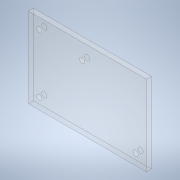
# Autodesk Inventor part: Template
Saved by Autodesk Inventor 2021 (Build 250183000, 183)
## iProperties
Created: 2021-05-20
Part Number: Template
Material: Polycarbonate, Clear
Document SubType Name: Modeling
Designer: maza168
Density: 1.2 g/cm^3
Appearance: Polycarbonate - Clear
Author: maza168
Autodesk Inventor part; units mm, degrees
ref_plane "YZ Plane" through (0, 0, 0) normal (1, 0, 0) x (0, 1, 0)
ref_plane "XZ Plane" through (0, 0, 0) normal (0, 1, 0) x (-1, 0, 0)
ref_plane "XY Plane" through (0, 0, 0) normal (0, 0, 1) x (1, 0, 0)
sketch "Sketch1" plane through (0, 0, 0) normal (0, 0, 1) x (1, 0, 0)
  line L0 (-110, 75) -> (110, 75)
  line L1 (110, 75) -> (110, -75)
  line L2 (110, -75) -> (-110, -75)
  line L3 (-110, -75) -> (-110, 75)
  line L4 (40, -10) -> (60, -10) construction
  line L5 (60, -10) -> (60, -30) construction
  line L6 (60, -30) -> (40, -30) construction
  line L7 (40, -30) -> (40, -10) construction
  line L8 (-67, 0) -> (-42, 0) construction
  line L9 (-42, 0) -> (-42, -30) construction
  line L10 (-42, -30) -> (-67, -30) construction
  line L11 (-67, -30) -> (-67, 0) construction
  circle A0 centre (-90, 55) radius 5
  circle A1 centre (-90, -55) radius 5
  circle A2 centre (90, -55) radius 5
  circle A3 centre (-10, 45) radius 5
  line L12 (-110, 75) -> (110, -75) construction
  line L13 (110, 75) -> (-110, -75) construction
  point P0 (0, 0)
  dimension "d0" = 220
  dimension "d1" = 150
  dimension "d2" = 110
  dimension "d3" = 75
  dimension "d4" = 20
  dimension "d5" = 20
  dimension "d6" = 10
  dimension "d7" = 40
  dimension "d8" = 10
  dimension "d9" = 90
  dimension "d10" = 55
  dimension "d11" = 10
  dimension "d12" = 10
  dimension "d13" = 10
  dimension "d14" = 55
  dimension "d15" = 42
  dimension "d16" = 30
  dimension "d17" = 25
  dimension "d18" = 0
  dimension "d19" = 90
  dimension "d20" = 45
  dimension "d21" = 10
  dimension "d22" = 90
  dimension "d23" = 55
  constraints: 28 end point, 6 parallel, 4 centre point, 3 horizontal, 3 perpendicular
  measures "d0" distance of L1.end L2.end
  measures "d1" distance of L2.end L0.start
  measures "d2" distance from line of point (0, 0) L3
  measures "d3" distance from line of point (0, 0) L0
  measures "d4" distance of L5.end L6.end
  measures "d5" distance of L4.end L5.end
  measures "d6" distance from line of L4 point (0, 0)
  measures "d7" distance from line of L7 point (0, 0)
  measures "d8" diameter of A0
  measures "d9" horizontal distance of point (0, 0) A0.centre
  measures "d10" vertical distance of point (0, 0) A0.centre
  measures "d11" diameter of A1
  measures "d12" diameter of A2
  measures "d13" diameter of A3
  measures "d14" vertical distance of point (0, 0) A1.centre
  measures "d15" distance from line of point (0, 0) L9
  measures "d16" distance of L10.end L8.start
  measures "d17" distance of L9.end L10.end
  measures "d18" distance from line of point (0, 0) L8
  measures "d19" horizontal distance of point (0, 0) A1.centre
  measures "d20" vertical distance of point (0, 0) A3.centre
  measures "d21" horizontal distance of point (0, 0) A3.centre
  measures "d22" horizontal distance of point (0, 0) A2.centre
  measures "d23" vertical distance of point (0, 0) A2.centre
extrude "Extrusion1" add sketch "Sketch1" along normal blind 9.4
body "Solid1"
